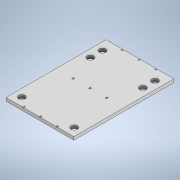
# Autodesk Inventor part: trucks
Saved by Autodesk Inventor 2021 (Build 250183000, 183)
## iProperties
Created: 2021-03-01
Part Number: trucks
Material: Generic
Document SubType Name: Modeling
Designer: Patrick
Density: 1 g/cm^3
Appearance: Default
Author: Patrick
Autodesk Inventor part; units mm, degrees
ref_plane "YZ Plane" through (0, 0, 0) normal (1, 0, 0) x (0, 1, 0)
ref_plane "XZ Plane" through (0, 0, 0) normal (0, 1, 0) x (-1, 0, 0)
ref_plane "XY Plane" through (0, 0, 0) normal (0, 0, 1) x (1, 0, 0)
sketch "Sketch1" plane through (0, 0, 0) normal (0, 1, 0) x (-1, 0, 0)
  line L0 (0, 0) -> (53.34, 0)
  line L1 (53.34, 0) -> (53.34, -78.74)
  line L2 (53.34, -78.74) -> (0, -78.74)
  line L3 (0, -78.74) -> (0, 0)
  circle A0 centre (47.3075, -6.35) radius 2.54
  circle A1 centre (47.3075, -60.325) radius 2.54
  circle A2 centre (47.3075, -69.85) radius 2.54
  circle A3 centre (6.0325, -6.35) radius 2.54
  circle A4 centre (6.0325, -60.325) radius 2.54
  circle A5 centre (6.0325, -69.85) radius 2.54
  line L4 (26.67, 0) -> (26.67, -78.74)
  dimension "d0" = 53.34
  dimension "d1" = 78.74
  dimension "d2" = 5.08
  dimension "d3" = 5.08
  dimension "d4" = 5.08
  dimension "d5" = 53.975
  dimension "d6" = 63.5
  dimension "d9" = 41.275
  dimension "d14" = 20.6375
  dimension "d16" = 6.35
  constraints: 10 end point, 6 centre point, 2 horizontal, 2 midpoint, 2 parallel, 1 perpendicular, 6 other
  measures "d0" distance between parallel lines of L3 L1
  measures "d1" distance between parallel lines of L0 L2
  measures "d2" diameter of A0
  measures "d3" diameter of A1
  measures "d4" diameter of A2
  measures "d5" distance of A1.centre A0.centre
  measures "d6" distance of A2.centre A0.centre
  measures "d9" distance of A0.centre A3.centre
  measures "d14" distance from line of L4 A3.centre
  measures "d16" distance from line of L0 A0.centre
extrude "Extrusion1" add sketch "Sketch1" along normal blind 2.54
sketch "Sketch2" plane through (0, 2.54, 0) normal (0, 1, 0) x (1, 0, 0)
  line L0 (-53.34, 0) -> (0, 0) projected
  line L1 (-53.34, 78.74) -> (-53.34, 0) projected
  line L2 (0, 78.74) -> (-53.34, 78.74) projected
  line L3 (0, 0) -> (0, 78.74) projected
  circle A0 centre (-6.0325, 6.35) radius 2.54 projected
  circle A1 centre (-6.0325, 60.325) radius 2.54 projected
  circle A2 centre (-6.0325, 69.85) radius 2.54 projected
  circle A3 centre (-47.3075, 69.85) radius 2.54 projected
  circle A4 centre (-47.3075, 60.325) radius 2.54 projected
  circle A5 centre (-47.3075, 6.35) radius 2.54 projected
  line L4 (-26.67, 0) -> (-26.67, 78.74)
  line L5 (0, 78.74) -> (-53.34, 78.74) projected
  line L6 (-26.67, 0) -> (-39.37, 0)
  line L7 (-39.37, 0) -> (-39.37, 78.74)
  line L8 (-39.37, 78.74) -> (-26.67, 78.74)
  line L9 (-26.67, 78.74) -> (-26.67, 0)
  line L10 (-26.67, 0) -> (-13.97, 0)
  line L11 (-13.97, 0) -> (-13.97, 78.74)
  line L12 (-13.97, 78.74) -> (-26.67, 78.74)
  line L13 (-26.67, 78.74) -> (-26.67, 0)
  line L14 (-39.37, 0) -> (-40.386, 0)
  line L15 (-40.386, 0) -> (-40.386, 78.74)
  line L16 (-40.386, 78.74) -> (-39.37, 78.74)
  line L17 (-39.37, 78.74) -> (-39.37, 0)
  line L18 (-26.67, 0) -> (-27.178, 0)
  line L19 (-27.178, 0) -> (-27.178, 78.74)
  line L20 (-27.178, 78.74) -> (-26.67, 78.74)
  line L21 (-26.67, 78.74) -> (-26.67, 0)
  line L22 (-53.34, 0) -> (0, 0) projected
  line L23 (-26.67, 78.74) -> (-26.162, 78.74)
  line L24 (-26.162, 78.74) -> (-26.162, 0)
  line L25 (-26.162, 0) -> (-26.67, 0)
  line L26 (-26.67, 0) -> (-26.67, 78.74)
  line L27 (-13.97, 0) -> (-12.954, 0)
  line L28 (-12.954, 0) -> (-12.954, 78.74)
  line L29 (-12.954, 78.74) -> (-13.97, 78.74)
  line L30 (-13.97, 78.74) -> (-13.97, 0)
  line L31 (-40.386, 0) -> (-12.954, 0)
  line L32 (-12.954, 0) -> (-12.954, 1.27)
  line L33 (-12.954, 1.27) -> (-40.386, 1.27)
  line L34 (-40.386, 1.27) -> (-40.386, 0)
  line L35 (-12.954, 78.74) -> (-40.386, 78.74)
  line L36 (-40.386, 78.74) -> (-40.386, 77.47)
  line L37 (-40.386, 77.47) -> (-12.954, 77.47)
  line L38 (-12.954, 77.47) -> (-12.954, 78.74)
  line L39 (-53.34, 39.37) -> (0, 39.37)
  line L40 (0, 0) -> (0, 78.74) projected
  line L41 (-40.386, 39.37) -> (-12.954, 39.37)
  line L42 (-12.954, 39.37) -> (-12.954, 40.005)
  line L43 (-12.954, 40.005) -> (-40.386, 40.005)
  line L44 (-40.386, 40.005) -> (-40.386, 39.37)
  line L45 (-40.386, 39.37) -> (-12.954, 39.37)
  line L46 (-12.954, 39.37) -> (-12.954, 38.735)
  line L47 (-12.954, 38.735) -> (-40.386, 38.735)
  line L48 (-40.386, 38.735) -> (-40.386, 39.37)
  line L49 (-40.386, 38.735) -> (-39.37, 38.735)
  line L50 (-39.37, 38.735) -> (-39.37, 39.37)
  line L51 (-39.37, 39.37) -> (-40.386, 39.37)
  line L52 (-40.386, 39.37) -> (-40.386, 38.735)
  point P0 (-13.97, 38.735)
  point P1 (-13.97, 40.005)
  point P2 (-27.178, 38.735)
  point P3 (-26.162, 38.735)
  point P4 (-26.162, 40.005)
  point P5 (-27.178, 40.005)
  point P6 (-13.97, 1.27)
  point P7 (-27.178, 1.27)
  point P8 (-26.162, 1.27)
  point P9 (-39.37, 1.27)
  point P10 (-13.97, 77.47)
  point P11 (-27.178, 77.47)
  point P12 (-26.162, 77.47)
  point P13 (-39.37, 77.47)
  point P14 (-39.37, 38.735)
  point P15 (-39.37, 40.005)
  dimension "d19" = 12.7
  dimension "d20" = 12.7
  dimension "d22" = 0.508
  dimension "d23" = 0.508
  dimension "d24" = 1.016
  dimension "d25" = 1.016
  dimension "d26" = 1.27
  dimension "d27" = 1.27
  dimension "d28" = 0.635
  dimension "d29" = 0.635
  constraints: 92 end point, 22 parallel, 11 horizontal, 11 perpendicular, 11 point on line, 6 midpoint, 2 other
  measures "d19" distance of L7.end L8.end
  measures "d20" distance of L12.end L11.end
  measures "d22" distance of L19.end L20.end
  measures "d23" distance of L24.end L25.end
  measures "d24" distance between parallel lines of L17 L15
  measures "d25" distance of L29.end L28.end
  measures "d26" distance between parallel lines of L33 L0
  measures "d27" distance between parallel lines of L2 L37
  measures "d28" distance between parallel lines of L43 L41
  measures "d29" distance between parallel lines of L39 L47
extrude "Extrusion2" cut sketch "Sketch2" against normal blind 0.5 contours L15 L33 L7 L0 | L39 L7 L47 L15 | L15 L43 L7 L39 | L19 L33 L4 L0 | L2 L7 L37 L15 | L4 L33 L24 L0 | L39 L4 L47 L19 | L19 L43 L4 L39 | L2 L4 L37 L19 | L39 L24 L47 L4 | L4 L43 L24 L39 | L11 L33 L28 L0 | L2 L24 L37 L4 | L39 L28 L47 L11 | L11 L43 L28 L39 | L2 L28 L37 L11
body "Solid1"
